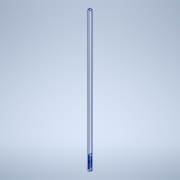
# Autodesk Inventor part: 12ｘ12_1
Saved by Autodesk Inventor 2020.3 (Build 243373000, 373)
## iProperties
Created: 2020-07-05
Part Number: 12ｘ12_1
Material: アルミニウム 6061
Document SubType Name: Modeling
Designer: totot
Density: 2.7 g/cm^3
Appearance: アルミニウム - フラット
Mass: 209.138 g
Surface Area: 1051.08 cm^2
Volume: 77.4586 cm^3
Author: totot
Autodesk Inventor part; units mm, degrees
ref_plane "YZ Plane" through (0, 0, 0) normal (1, 0, 0) x (0, 1, 0)
ref_plane "XZ Plane" through (0, 0, 0) normal (0, 1, 0) x (-1, 0, 0)
ref_plane "XY Plane" through (0, 0, 0) normal (0, 0, 1) x (1, 0, 0)
sketch "スケッチ1" plane through (0, 0, 0) normal (0, 1, 0) x (-1, 0, 0)
  line L0 (0, 0) -> (-15, 0)
  line L1 (-15, 0) -> (-15, -15)
  line L2 (-15, -15) -> (0, -15)
  line L3 (0, -15) -> (0, 0)
  line L4 (-1.5, -1.5) -> (-13.5, -1.5)
  line L5 (-13.5, -1.5) -> (-13.5, -13.5)
  line L6 (-13.5, -13.5) -> (-1.5, -13.5)
  line L7 (-1.5, -13.5) -> (-1.5, -1.5)
  dimension "d0" = 15
  dimension "d1" = 15
  dimension "d2" = 12
  dimension "d3" = 12
  dimension "d4" = 1.5
  dimension "d5" = 1.5
  constraints: 16 end point, 4 parallel, 2 horizontal, 2 perpendicular
  measures "d0" distance of L2.end L1.end
  measures "d1" distance of L1.end L0.end
  measures "d2" distance of L6.end L5.end
  measures "d3" distance of L6.end L4.start
  measures "d4" distance between parallel lines of L7 L3
  measures "d5" distance between parallel lines of L2 L6
extrude "押し出し1" add sketch "スケッチ1" along normal blind 1000
sketch "スケッチ3" plane through (15, 0, 0) normal (0, 0, 1) x (1, 0, 0)
  line L0 (-15, 0) -> (-15, 1000) projected
  line L1 (-15, 0) -> (0, 0) projected
  point P0 (-7.5, 7.5)
  point P1 (-7.5, 107.5)
  dimension "d8" = 7.5
  dimension "d9" = 7.5
  dimension "d10" = 7.5
  dimension "d11" = 100
  measures "d8" distance from line of point (-7.5, 7.5) L0
  measures "d9" distance from line of point (-7.5, 107.5) L0
  measures "d10" distance from line of point (-7.5, 7.5) L1
  measures "d11" distance of point (-7.5, 107.5) point (-7.5, 7.5)
hole "穴1" at (7.5, 7.5, 0) at (7.5, 107.5, 0) direction (0, 0, -1) diameter 3 end through all
sketch "スケッチ4" plane through (0, 0, 0) normal (-1, 0, 0) x (0, 0, 1)
  line L0 (-15, 0) -> (0, 0) projected
  line L1 (-15, 0) -> (-15, 1000) projected
  point P0 (-7.5, 16.5)
  point P1 (-7.5, 98.5)
  dimension "d19" = 16.5
  dimension "d20" = 7.5
  dimension "d21" = 7.5
  dimension "d22" = 82
  measures "d19" distance from line of point (-7.5, 16.5) L0
  measures "d20" distance from line of point (-7.5, 16.5) L1
  measures "d21" distance from line of point (-7.5, 98.5) L1
  measures "d22" distance of point (-7.5, 98.5) point (-7.5, 16.5)
hole "穴2" at (0, 16.5, -7.5) at (0, 98.5, -7.5) direction (1, 0, 0) diameter 3 end through all
sketch "スケッチ5" plane through (15, 0, -15) normal (1, 0, 0) x (0, 0, -1)
  line L0 (0, 0) -> (0, 1000) projected
  line L1 (-15, 1000) -> (0, 1000) projected
  point P0 (-15, 0)
  point P1 (-7.5, 992.5)
  dimension "d30" = 7.5
  dimension "d31" = 7.5
  measures "d30" distance from line of L0 point (-7.5, 992.5)
  measures "d31" distance from line of point (-7.5, 992.5) L1
hole "穴3" at (15, 992.5, -7.5) direction (-1, 0, 0) diameter 3 end through all
sketch "スケッチ6" plane through (15, 0, 0) normal (0, 0, 1) x (1, 0, 0)
  circle A0 centre (-7.5, 7.5) radius 1.5 projected
  circle A1 centre (-7.5, 107.5) radius 1.5 projected
  line L0 (-7.5, 7.5) -> (-7.5, 107.5)
  point P0 (-15, 0)
  point P1 (-7.5, 17.5)
  point P2 (-7.5, 27.5)
  point P3 (-7.5, 37.5)
  point P4 (-7.5, 47.5)
  point P5 (-7.5, 57.5)
  point P6 (-7.5, 67.5)
  point P7 (-7.5, 77.5)
  point P8 (-7.5, 87.5)
  point P9 (-7.5, 97.5)
  dimension "d39" = 100
  dimension "d40" = 10
  dimension "d43" = 10
  constraints: 2 end point, 2 vertical, 1 point on line, 8 other
  measures "d39" distance of L0.start L0.end
  measures "d40" distance of point (-7.5, 17.5) L0.start
  measures "d43" distance of point (-7.5, 17.5) point (-7.5, 27.5)
hole "穴4" at (7.5, 17.5, 0) at (7.5, 27.5, 0) at (7.5, 37.5, 0) at (7.5, 47.5, 0) at (7.5, 57.5, 0) at (7.5, 67.5, 0) at (7.5, 77.5, 0) at (7.5, 87.5, 0) at (7.5, 97.5, 0) direction (0, 0, -1) diameter 9 end through all
sketch "スケッチ7" plane through (15, 0, -15) normal (1, 0, 0) x (0, 0, -1)
  circle A0 centre (-7.5, 16.5) radius 1.5 projected
  circle A1 centre (-7.5, 98.5) radius 1.5 projected
  line L0 (-7.5, 16.5) -> (-7.5, 98.5)
  point P0 (-15, 0)
  point P1 (-7.5, 26.75)
  point P2 (-7.5, 37)
  point P3 (-7.5, 47.25)
  point P4 (-7.5, 57.5)
  point P5 (-7.5, 67.75)
  point P6 (-7.5, 78)
  point P7 (-7.5, 88.25)
  dimension "d55" = 82
  dimension "d56" = 10.25
  dimension "d59" = 10.25
  constraints: 2 end point, 2 vertical, 1 point on line, 6 other
  measures "d55" distance of L0.start L0.end
  measures "d56" distance of L0.start point (-7.5, 26.75)
  measures "d59" distance of point (-7.5, 26.75) point (-7.5, 37)
hole "穴5" at (15, 26.75, -7.5) at (15, 37, -7.5) at (15, 47.25, -7.5) at (15, 57.5, -7.5) at (15, 67.75, -7.5) at (15, 78, -7.5) at (15, 88.25, -7.5) direction (-1, 0, 0) diameter 9 end through all
sketch "スケッチ8" plane through (15, 0, -15) normal (1, 0, 0) x (0, 0, -1)
  line L0 (-15, 0) -> (-15, 1000) projected
  line L1 (-15, 0) -> (0, 0) projected
  circle A0 centre (-7.5, 98.5) radius 1.5 projected
  point P0 (-7.5, 7.5)
  point P1 (-7.5, 107.5)
  dimension "d71" = 7.5
  dimension "d72" = 7.5
  dimension "d73" = 7.5
  dimension "d74" = 9
  measures "d71" distance from line of point (-7.5, 7.5) L0
  measures "d72" distance from line of point (-7.5, 107.5) L0
  measures "d73" distance from line of point (-7.5, 7.5) L1
  measures "d74" distance of point (-7.5, 107.5) A0.centre
hole "穴6" at (15, 7.5, -7.5) at (15, 107.5, -7.5) direction (-1, 0, 0) diameter 9 end through all
equation "\"d3\" = d2"
equation "\"d4\" = d5"
equation "\"d9\" = d8"
equation "\"d10\" = d8"
equation "\"d21\" = d20"
equation "\"d31\" = d30"
equation "\"d40\" = 0.1 * d39"
equation "\"d56\" = 0.125 * d55"
equation "\"d59\" = d56"
equation "\"d72\" = d71"
equation "\"d73\" = d71"
